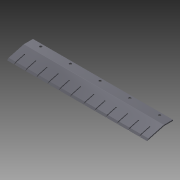
# Autodesk Inventor part: Cuña
Saved by Autodesk Inventor 2014 (Build 180170000, 170)
## iProperties
Created: 2014-01-28
Part Number: Cuña
Material: Acero dulce
Document SubType Name: Chapa
Designer: VICTOR
Mass: 83.5459 g
Surface Area: 157.543 cm^2
Volume: 10.6292 cm^3
Density: 7.86 g/cm^3
Sheet Metal Rule: Por defecto_mm
Project: ROBOT SUMO
Description: CUÑA
Flat Pattern Width: 3.8 cm
Flat Pattern Length: 20 cm
Flat Pattern Area: 76 cm^2
Sheet Metal Width: 38,000 mm
Sheet Metal Length: 200,000 mm
Sheet Metal Area: 7600,000 mm^2
Appearance: Acero - Pulido
Author: Usuario
Revision Number: 1
Autodesk Inventor part; units mm, degrees
ref_plane "YZ Plane" through (0, 0, 0) normal (1, 0, 0) x (0, 1, 0)
ref_plane "XZ Plane" through (0, 0, 0) normal (0, 1, 0) x (-1, 0, 0)
ref_plane "XY Plane" through (0, 0, 0) normal (0, 0, 1) x (1, 0, 0)
sketch "Boceto1" plane through (0, 0, 0) normal (0, 0, 1) x (1, 0, 0)
  line L0 (100, 13) -> (-100, 13)
  line L1 (-100, 13) -> (-100, -25)
  line L2 (-100, -25) -> (100, -25)
  line L3 (100, -25) -> (100, 13)
  point P0 (0, 0)
  dimension "d0" = 100
  dimension "d1" = 200
  dimension "d2" = 38
  dimension "d3" = 13
  measures "d0" distance from line of point (0, 0) L3
  measures "d1" distance of L1.end L2.end
  measures "d2" distance of L0.end L1.end
  measures "d3" distance from line of L0 point (0, 0)
extrude "Placa1" add sketch "Boceto1" along normal blind 1.5
sketch "Boceto2" plane through (0, 0, 1.5) normal (0, 0, 1) x (1, 0, 0)
  line L0 (100, 13) -> (100, -25) projected
  line L1 (-100, -25) -> (-100, 13) projected
  line L2 (100, -25) -> (-100, -25) projected
  line L3 (-100, 0) -> (100, 0)
  point P0 (0, 0)
  dimension "d5" = 25
  constraints: 2 end point, 2 point on line, 1 perpendicular
  measures "d5" distance between parallel lines of L2 L3
fold "Pliegue1" angle 15 bend radius 1 thickness 1.5 k factor 0.44 line from (-100, 0, 1.5) to (100, 0, 1.5) line at bend end moving side (0, -1, 0) folds toward (0, 0, -1)
sketch "Boceto3" plane through (-100, -24.3606, -5.0557) normal (0, -0.258819, 0.9659258) x (1, 0, 0)
  line L0 (0, 0) -> (0, 25) projected
  line L1 (200, 25) -> (200, 0) projected
  line L2 (190, 0) -> (189, 0)
  line L3 (189, 0) -> (189, 14.441)
  line L4 (190, 14.441) -> (190, 0)
  arc A0 (190, 14.441) -> (189, 14.441) centre (189.5, 15) ccw
  line L5 (11, 0) -> (10, 0)
  line L6 (10, 0) -> (10, 14.441)
  line L7 (11, 14.441) -> (11, 0)
  arc A1 (11, 14.441) -> (10, 14.441) centre (10.5, 15) ccw
  line L8 (174, 0) -> (173, 0)
  line L9 (173, 0) -> (173, 14.441)
  line L10 (174, 14.441) -> (174, 0)
  arc A2 (174, 14.441) -> (173, 14.441) centre (173.5, 15) ccw
  line L11 (27, 0) -> (26, 0)
  line L12 (26, 0) -> (26, 14.441)
  line L13 (27, 14.441) -> (27, 0)
  arc A3 (27, 14.441) -> (26, 14.441) centre (26.5, 15) ccw
  line L14 (43, 14.441) -> (43, 0)
  line L15 (43, 0) -> (42, 0)
  line L16 (42, 0) -> (42, 14.441)
  arc A4 (43, 14.441) -> (42, 14.441) centre (42.5, 15) ccw
  line L17 (157, 0) -> (157, 14.441)
  line L18 (158, 0) -> (157, 0)
  line L19 (158, 14.441) -> (158, 0)
  arc A5 (158, 14.441) -> (157, 14.441) centre (157.5, 15) ccw
  line L20 (59, 0) -> (58, 0)
  line L21 (58, 0) -> (58, 14.441)
  line L22 (59, 14.441) -> (59, 0)
  arc A6 (59, 14.441) -> (58, 14.441) centre (58.5, 15) ccw
  line L23 (75, 14.441) -> (75, 0)
  line L24 (75, 0) -> (74, 0)
  line L25 (74, 0) -> (74, 14.441)
  arc A7 (75, 14.441) -> (74, 14.441) centre (74.5, 15) ccw
  line L26 (91, 14.441) -> (91, 0)
  line L27 (90, 0) -> (90, 14.441)
  line L28 (91, 0) -> (90, 0)
  arc A8 (91, 14.441) -> (90, 14.441) centre (90.5, 15) ccw
  line L29 (142, 0) -> (141, 0)
  line L30 (141, 0) -> (141, 14.441)
  line L31 (142, 14.441) -> (142, 0)
  arc A9 (142, 14.441) -> (141, 14.441) centre (141.5, 15) ccw
  line L32 (125, 0) -> (125, 14.441)
  line L33 (126, 0) -> (125, 0)
  line L34 (126, 14.441) -> (126, 0)
  arc A10 (126, 14.441) -> (125, 14.441) centre (125.5, 15) ccw
  line L35 (109, 0) -> (109, 14.441)
  line L36 (110, 14.441) -> (110, 0)
  arc A11 (110, 14.441) -> (109, 14.441) centre (109.5, 15) ccw
  line L37 (110, 0) -> (109, 0)
  line L38 (200, 0) -> (0, 0) projected
  dimension "d12" = 1
  dimension "d13" = 1.5
  dimension "d14" = 10
  dimension "d16" = 1
  dimension "d17" = 1.5
  dimension "d18" = 15
  dimension "d19" = 10
  dimension "d20" = 1
  dimension "d21" = 1.5
  dimension "d23" = 1
  dimension "d24" = 1.5
  dimension "d25" = 15
  dimension "d26" = 15
  dimension "d27" = 15
  dimension "d28" = 1
  dimension "d29" = 1.5
  dimension "d31" = 15
  dimension "d32" = 1
  dimension "d33" = 1.5
  dimension "d35" = 15
  dimension "d38" = 1
  dimension "d39" = 1.5
  dimension "d41" = 1
  dimension "d42" = 1.5
  dimension "d44" = 15
  dimension "d45" = 1
  dimension "d46" = 1.5
  dimension "d48" = 15
  dimension "d49" = 15
  dimension "d50" = 1
  dimension "d51" = 1.5
  dimension "d53" = 1
  dimension "d54" = 1.5
  dimension "d56" = 15
  dimension "d57" = 1
  dimension "d58" = 1.5
  dimension "d60" = 15
  dimension "d61" = 15
  dimension "d65" = 15
  dimension "d66" = 15
  dimension "d67" = 15
  dimension "d68" = 15
  dimension "d69" = 15
  dimension "d70" = 15
  dimension "d71" = 15
  dimension "d72" = 15
  dimension "d73" = 15
  dimension "d74" = 15
  constraints: 72 end point, 24 point on circle, 12 centre point, 12 horizontal, 12 parallel, 12 perpendicular, 1 collinear
  measures "d12" distance of L2.start L2.end
  measures "d13" diameter of A0
  measures "d14" distance between parallel lines of L1 L4
  measures "d16" distance of L5.start L5.end
  measures "d17" diameter of A1
  measures "d18" distance from line of A1.centre L5
  measures "d19" distance between parallel lines of L0 L6
  measures "d20" distance of L8.start L9.start
  measures "d21" diameter of A2
  measures "d23" distance of L13.end L11.end
  measures "d24" diameter of A3
  measures "d25" distance from line of A3.centre L11
  measures "d26" distance between parallel lines of L10 L3
  measures "d27" distance between parallel lines of L12 L7
  measures "d28" distance of L14.end L16.start
  measures "d29" diameter of A4
  measures "d31" distance between parallel lines of L16 L13
  measures "d32" distance of L19.end L17.start
  measures "d33" diameter of A5
  measures "d35" distance between parallel lines of L9 L19
  measures "d38" distance of L22.end L20.end
  measures "d39" diameter of A6
  measures "d41" distance of L23.end L24.end
  measures "d42" diameter of A7
  measures "d44" distance between parallel lines of L25 L22
  measures "d45" distance of L26.end L27.start
  measures "d46" diameter of A8
  measures "d48" distance between parallel lines of L27 L23
  measures "d49" distance between parallel lines of L21 L14
  measures "d50" distance of L31.end L30.start
  measures "d51" diameter of A9
  measures "d53" distance of L33.start L32.start
  measures "d54" diameter of A10
  measures "d56" distance between parallel lines of L34 L30
  measures "d57" distance of L36.end L35.start
  measures "d58" diameter of A11
  measures "d60" distance between parallel lines of L32 L36
  measures "d61" distance between parallel lines of L17 L31
  measures "d65" distance from line of L38 A4.centre
  measures "d66" distance from line of L38 A6.centre
  measures "d67" distance from line of L38 A7.centre
  measures "d68" distance from line of L38 A8.centre
  measures "d69" distance from line of L38 A11.centre
  measures "d70" distance from line of L38 A10.centre
  measures "d71" distance from line of L38 A9.centre
  measures "d72" distance from line of L38 A5.centre
  measures "d73" distance from line of L38 A2.centre
  measures "d74" distance from line of L38 A0.centre
extrude "Cortar2" cut sketch "Boceto3" against normal blind 1.5
sketch "Boceto5" plane through (100, -23.9724, -6.5046) normal (1, 0, 0) x (0, 0.258819, -0.9659258)
  line L0 (0, 0) -> (-1.5, 0) projected
  line L1 (0, 0) -> (-1.5, 2.5981)
  line L2 (-1.5, 0) -> (-1.5, 2.5981)
  point P0 (-0.0784, 24.839)
  dimension "d105" = 60
  constraints: 4 end point, 1 perpendicular
  measures "d105" angle of L0 L1
extrude "Extrusión1" cut sketch "Boceto5" against normal through all
sketch "Boceto6" plane through (0, 0, 1.5) normal (0, 0, 1) x (1, 0, 0)
  point P0 (42.5, 9)
  point P1 (-42.5, 9)
  point P2 (-85, 9)
  point P3 (0, 9)
  point P4 (85, 9)
hole "Hole3" at (42.5, 9, 1.5) at (-42.5, 9, 1.5) at (-85, 9, 1.5) at (0, 9, 1.5) at (85, 9, 1.5) direction (0, 0, -1) diameter 3.4 depth 1.5
equation "\"d6\" = Anchura_desahogo_plegado"
equation "\"d7\" = Profundidad_desahogo_plegado"
equation "\"d8\" = Remanente_mínimo"
equation "\"d9\" = Radio_pliegue"
equation "\"d62\" = Grosor"
equation "\"Radio_pliegue\" = Grosor"
equation "\"Anchura_desahogo_plegado\" = Grosor"
equation "\"Profundidad_desahogo_plegado\" = 0.5 * Grosor"
equation "\"Tamaño_destalonado\" = 4 * Grosor"
equation "\"Remanente_mínimo\" = 2 * Grosor"
equation "\"Radiodetransición\" = Radio_pliegue"
equation "\"Tamaño_de_radio_de_Jacobi\" = Radio_pliegue"
equation "\"TamañoSeparación\" = Grosor"
equation "\"d4\" = Radio_pliegue"
equation "\"Grosor\" = 1.5"
